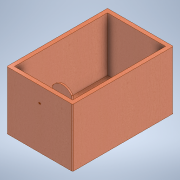
# Autodesk Inventor part: BoxDark
Saved by Autodesk Inventor 2022.2 (Build 262287010, 287A)
## iProperties
Created: 2022-03-17
Part Number: BoxDark
Material: Genérico
Document SubType Name: Modeling
Designer: mabel
Density: 1 g/cm^3
Appearance: Nogal - Natural pulido
Author: mabel
Autodesk Inventor part; units mm, degrees
ref_plane "YZ Plane" through (0, 0, 0) normal (1, 0, 0) x (0, 1, 0)
ref_plane "XZ Plane" through (0, 0, 0) normal (0, 1, 0) x (-1, 0, 0)
ref_plane "XY Plane" through (0, 0, 0) normal (0, 0, 1) x (1, 0, 0)
sketch "Boceto1" plane through (0, 0, 0) normal (0, 1, 0) x (-1, 0, 0)
  line L0 (-85, -130) -> (85, -130)
  line L1 (85, -130) -> (85, 130)
  line L2 (85, 130) -> (-85, 130)
  line L3 (-85, 130) -> (-85, -130)
  line L4 (-85, -130) -> (85, 130) construction
  line L5 (85, -130) -> (-85, 130) construction
  line L6 (75, 120) -> (75, -120)
  line L7 (75, -120) -> (-75, -120)
  line L8 (-75, -120) -> (-75, 120)
  line L9 (-75, 120) -> (75, 120)
  point P0 (0, 0)
  point P1 (0, -120)
  point P2 (0, 120)
  point P3 (0, 0)
  dimension "d0" = 170
  dimension "d1" = 260
  dimension "d10" = 10
  constraints: 20 end point, 5 midpoint, 4 parallel, 2 perpendicular, 1 horizontal, 3 other
  measures "d0" distance of L2.end L1.end
  measures "d1" distance of L1.end L0.end
  measures "d10" distance between parallel lines of L1 L6
extrude "Extrusión1" add sketch "Boceto1" along normal blind 150
extrude "Extrusión3" add sketch "Boceto1" along normal blind 10 contours L6 L7 L8 L9
sketch "Boceto4" plane through (0, 10, 0) normal (0, 1, 0) x (1, 0, 0)
  circle A0 centre (0, 4.19) radius 3.75
  line L0 (85, 130) -> (-85, 130) projected
  circle A1 centre (0, 4.19) radius 3.35
  circle A2 centre (0, 4.19) radius 1.5
  line L1 (-85, -130) -> (85, -130) projected
  line L2 (75, -120) -> (-75, -120) construction
  line L3 (0, -120) -> (0, -70) construction
  point P0 (0, 0)
  dimension "d15" = 7.5
  dimension "d17" = 0.4
  dimension "d20" = 3
  dimension "d23" = 134.19
  dimension "d36" = 50
  constraints: 3 centre point, 2 end point, 1 coincident, 1 midpoint, 1 vertical
  measures "d15" diameter of A0
  measures "d17" radial gap between concentric circles of A0 A1
  measures "d20" diameter of A2
  measures "d23" distance from line of A0.centre L1
  measures "d36" distance of L3.start L3.end
extrude "Extrusión4" add sketch "Boceto4" along normal blind 21 contours A0
extrude "Extrusión5" cut sketch "Boceto4" against normal blind 10 contours A2
sketch "Boceto7" plane through (0, 10, 0) normal (0, 1, 0) x (1, 0, 0)
  circle A0 centre (0, 4.19) radius 1.5 construction
  line L0 (0, 4.19) -> (-17.5, 4.19) construction
  line L1 (-17.5, -27.68) -> (-4.5, -27.68)
  line L2 (-4.5, -27.68) -> (-4.5, -22.68)
  line L3 (-4.5, -22.68) -> (-17.5, -22.68)
  line L4 (-17.5, -22.68) -> (-17.5, -27.68)
  circle A1 centre (0, 4.19) radius 1.5 construction
  line L5 (0, 4.19) -> (0, -27.68) construction
  line L6 (0, -27.68) -> (-11, -27.68) construction
  line L7 (17.5, -27.68) -> (4.5, -27.68)
  line L8 (4.5, -27.68) -> (4.5, -22.68)
  line L9 (4.5, -22.68) -> (17.5, -22.68)
  line L10 (17.5, -22.68) -> (17.5, -27.68)
  line L11 (-17.5, 36.06) -> (-4.5, 36.06)
  line L12 (-4.5, 36.06) -> (-4.5, 31.06)
  line L13 (-4.5, 31.06) -> (-17.5, 31.06)
  line L14 (-17.5, 31.06) -> (-17.5, 36.06)
  line L15 (17.5, 31.06) -> (17.5, 36.06)
  line L16 (17.5, 36.06) -> (4.5, 36.06)
  line L17 (4.5, 31.06) -> (17.5, 31.06)
  line L18 (4.5, 36.06) -> (4.5, 31.06)
  line L19 (-4.5, -27.68) -> (-5.1934, -27.68)
  line L20 (75, -120) -> (-75, -120) construction
  line L21 (0, -120) -> (0, -70) construction
  line L22 (0, -70) -> (-19.0745, -70) construction
  line L23 (25, -68) -> (-25, -68)
  line L24 (-25, -68) -> (-25, -72)
  line L25 (-25, -72) -> (25, -72)
  line L26 (25, -72) -> (25, -68)
  line L27 (25, -68) -> (-25, -72) construction
  line L28 (-25, -68) -> (25, -72) construction
  line L29 (-23.5, -70.5) -> (-23.5, -69.5)
  line L30 (-23.5, -69.5) -> (23.5, -69.5)
  line L31 (23.5, -69.5) -> (23.5, -70.5)
  line L32 (23.5, -70.5) -> (-23.5, -70.5)
  point P0 (0, 0)
  dimension "d43" = 31.87
  dimension "d44" = 50
  dimension "d45" = 50
  dimension "d46" = 4
  dimension "d47" = 1.5
  constraints: 64 end point, 6 parallel, 5 perpendicular, 3 horizontal, 3 midpoint, 2 point on line, 2 vertical, 3 other
  measures "d43" distance of L5.start L5.end
  measures "d44" distance of L21.start L21.end
  measures "d45" distance of L25.end L24.end
  measures "d46" distance of L24.end L23.end
  measures "d47" distance between parallel lines of L24 L29
extrude "Extrusión7" cut sketch "Boceto7" against normal blind 5 contours L4 L3 L2 L1 | L7 L8 L9 L10 | L11 L12 L13 L14 | L17 L18 L16 L15
sketch "Boceto8" plane through (75, 150, 120) normal (0, 0, -1) x (-1, 0, 0)
  line L0 (0, -140) -> (150, -140) construction
  line L1 (75, -140) -> (75, -40) construction
  circle A0 centre (75, -40) radius 5
  circle A1 centre (75, -40) radius 1.5
  point P0 (75, -150)
  dimension "d37" = 100
  dimension "d38" = 10
  dimension "d75" = 3
  constraints: 2 centre point, 2 end point, 1 coincident, 1 midpoint, 1 vertical
  measures "d37" distance of L1.start L1.end
  measures "d38" diameter of A0
  measures "d75" diameter of A1
extrude "Extrusión9" add sketch "Boceto7" along normal blind 100 contours L26 L25 L24 L23
sketch "Boceto9" plane through (-25, 10, 72) normal (0, 0, 1) x (1, 0, 0)
  line L0 (0, 100) -> (25, 85.5662)
  line L1 (0, 100) -> (57.416, 100) construction
  line L2 (50, 100) -> (25, 85.5662)
  line L3 (50, 100) -> (104.7106, 100) construction
  arc A0 (48.8838, 99.3556) -> (1.1162, 99.3556) centre (25, 85.5662) ccw
  line L4 (0, 100) -> (1.5, 100)
  line L5 (0, 100) -> (50, 100) projected
  line L6 (50, 100) -> (48.5, 100)
  point P0 (25, -10)
  constraints: 12 end point, 4 point on circle, 3 point on line, 2 horizontal, 1 centre point, 1 coincident, 1 collinear
extrude "Extrusión11" add sketch "Boceto9" against normal blind 4 contours A0 L5 L2 L0 | A0 L5
extrude "Extrusión12" cut sketch "Boceto9" against normal blind 4 contours A0 L5 L2 L0 | A0 L5
extrude "Extrusión13" cut sketch "Boceto9" against normal blind 4 contours L4 A0 L0
extrude "Extrusión14" cut sketch "Boceto9" against normal blind 4 contours L5 L2 A0
extrude "Extrusión15" add sketch "Boceto9" against normal blind 4 contours A0 L5
extrude "Extrusión16" add sketch "Boceto9" against normal blind 4 contours A0 L5 L2 L0
fillet "Empalme1" radius 2 4 edges at (85, 75, 130) (-85, 75, 130) (85, 75, -130) (-85, 75, -130)
extrude "Extrusión17" add sketch "Boceto8" along normal blind 1 contours A1
sketch "Boceto16" plane through (-83, 0, 130) normal (0, 0, 1) x (1, 0, 0)
  circle A0 centre (83, 110) radius 1.5 projected
  circle A1 centre (83, 110) radius 2
  line L0 (82.8, 109.425) -> (80.2, 109.425)
  line L1 (80.2, 109.425) -> (80.2, 110.575)
  line L2 (80.2, 110.575) -> (82.8, 110.575)
  line L3 (82.8, 110.575) -> (82.8, 109.425)
  circle A2 centre (83, 110) radius 1.5 projected
  line L4 (82.8, 109.425) -> (80.2, 110.575) construction
  line L5 (80.2, 109.425) -> (82.8, 110.575) construction
  line L6 (85.8, 109.425) -> (83.2, 109.425)
  line L7 (83.2, 109.425) -> (83.2, 110.575)
  line L8 (83.2, 110.575) -> (85.8, 110.575)
  line L9 (85.8, 110.575) -> (85.8, 109.425)
  line L10 (85.8, 109.425) -> (83.2, 110.575) construction
  line L11 (83.2, 109.425) -> (85.8, 110.575) construction
  point P0 (83, 0)
  point P1 (81.5, 110)
  point P2 (84.5, 110)
  dimension "d78" = 4
  dimension "d81" = 2.6
  dimension "d82" = 1.15
  dimension "d83" = 2.6
  constraints: 24 end point, 4 midpoint, 4 parallel, 2 horizontal, 2 perpendicular, 2 point on circle, 1 centre point, 1 coincident
  measures "d78" diameter of A1
  measures "d81" distance of L1.end L2.end
  measures "d82" distance of L0.end L1.end
  measures "d83" distance of L7.end L8.end
extrude "Extrusión18" cut sketch "Boceto16" against normal blind 1 contours A0 L8 A1 L6 | A0 L2 A1 L8 | L6 A1 L0 A0 | A0 L0 A1 L2
extrude "Extrusión19" add sketch "Boceto16" along normal blind 0.25 contours A0 L6 L7 L8 | A0 L8 A1 L6 | L2 L3 L0 A0 | A0 L0 A1 L2 | L8 L9 L6 A1 | A1 L0 L1 L2
